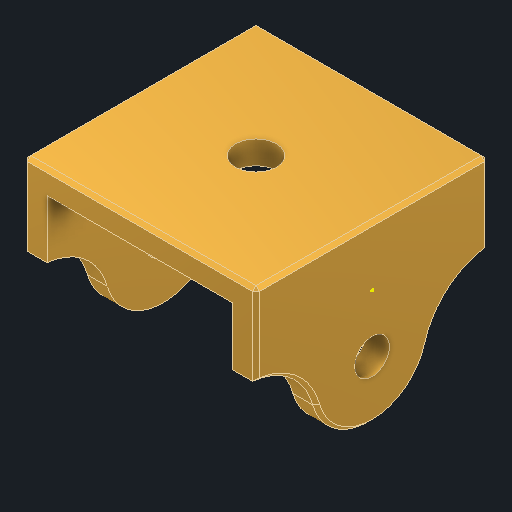
# Autodesk Inventor part: Ball Track Mounting Plate
Saved by Autodesk Inventor 2027.1 (Build 311270010, 270A)
## iProperties
Created: 2025-09-16
Material: Brass, Soft Yellow
Document SubType Name: Modeling
Designer: SD
Density: 8.47 g/cm^3
Appearance: Brass - Satin
Mass: 12.4367 g
Surface Area: 17.3579 cm^2
Volume: 1.46832 cm^3
Project: Automatic Tea Steeping mechanism
Part Number: Ball Track Mounting Plate
d6: 2.000 mm
Length: 20.000 mm
Thickness: 10.000 mm
Width: 20.000 mm
BOM-Mass: 0.01244
BOM-Area: 0.002
Procurement: Fabricate - 2nd round
Build Stage: 3
Preferred Material: C36000 Brass
Author: SD
Title: Ball Track Mounting Plate
Autodesk Inventor part; units mm, degrees
ref_plane "YZ Plane" through (0, 0, 0) normal (1, 0, 0) x (0, 1, 0)
ref_plane "XZ Plane" through (0, 0, 0) normal (0, 1, 0) x (-1, 0, 0)
ref_plane "XY Plane" through (0, 0, 0) normal (0, 0, 1) x (1, 0, 0)
sketch "Sketch1" plane through (0, 0, 0) normal (0, 0, 1) x (1, 0, 0)
  line L0 (-10, 5) -> (10, 5)
  line L1 (10, 5) -> (10, -5)
  line L2 (10, -5) -> (-10, -5)
  line L3 (-10, -5) -> (-10, 5)
  line L4 (-10, 5) -> (10, -5) construction
  line L5 (10, 5) -> (-10, -5) construction
  point P0 (0, 0)
  constraints: 12 end point, 4 parallel, 2 midpoint, 1 horizontal, 1 perpendicular
extrude "Extrusion1" add sketch "Sketch1" along normal mid plane 20
sketch "Sketch3" plane through (10, -5, 10) normal (1, 0, 0) x (0, 0, -1)
  point P0 (10, 5)
sketch "Sketch4" plane through (10, -5, 10) normal (1, 0, 0) x (0, 0, -1)
  line L0 (0, 0) -> (20, 0) projected
  arc A0 (5, 0) -> (15, 0) centre (10, 0) ccw
  point P0 (10, 5)
  dimension "d9" = 10
  constraints: 2 point on circle, 2 point on line, 1 centre point, 1 midpoint
  measures "d9" diameter of A0
extrude "Extrusion3" add sketch "Sketch4" against normal up to surface (20 mm away)
sketch "Sketch2" plane through (0, 0, 10) normal (0, 0, 1) x (1, 0, 0)
  line L0 (-8, -16.4616) -> (8, -16.4616)
  line L1 (8, -16.4616) -> (8, 3)
  line L2 (8, 3) -> (-8, 3)
  line L3 (-8, 3) -> (-8, -16.4616)
  line L4 (-10, 5) -> (-10, -5) projected
  line L5 (10, -5) -> (10, 5) projected
  line L6 (10, 5) -> (-10, 5) projected
  point P0 (0, 0)
  dimension "d4" = 2
  dimension "d5" = 2
  dimension "d6" = 2
  constraints: 8 end point, 2 parallel, 1 horizontal, 1 perpendicular
  measures "d4" distance between parallel lines of L3 L4
  measures "d5" distance between parallel lines of L5 L1
  measures "d6" distance between parallel lines of L2 L6
extrude "Extrusion2" cut sketch "Sketch2" against normal blind 30
sketch "Sketch5" plane through (10, -5, 10) normal (1, 0, 0) x (0, 0, -1)
  line L0 (0, 8) -> (0, 0) projected
  line L1 (5, 0) -> (0, 0) projected
  line L2 (0, 3) -> (5, 3)
  line L3 (5, 3) -> (5, 0)
  line L4 (5, 0) -> (0, 0)
  line L5 (0, 0) -> (0, 3)
  arc A0 (5, 0) -> (15, 0) centre (10, 0) ccw projected
  line L6 (20, 10) -> (20, 0) projected
  line L7 (15, 0) -> (20, 0)
  line L8 (20, 0) -> (20, 3)
  line L9 (20, 3) -> (15, 3)
  line L10 (15, 3) -> (15, 0)
  point P0 (10, 5)
  dimension "d12" = 3
  constraints: 16 end point, 5 parallel, 2 horizontal, 2 perpendicular, 2 point on line
  measures "d12" distance between parallel lines of L1 L2
extrude "Extrusion4" cut sketch "Sketch5" against normal blind 30
fillet "Fillet1" radius 6 4 edges at (9, -2, 5) (9, -2, -5) (-9, -2, 5) (-9, -2, -5)
chamfer "Chamfer1" distance 0.3 angle 45 14 edges at (0, 5, 10) (10, 5, 0) (0, 5, -10) (-10, 5, 0) (-10, 1.5, 10) (10, 1.5, 10) (10, 1.5, -10) (-10, 1.5, -10) (-10, -3.3741, -6.7351) (-10, -10, 0) (-10, -3.3741, 6.7351) (10, -3.3741, -6.7351) (10, -10, 0) (10, -3.3741, 6.7351)
sketch "Sketch6" plane through (-10, -4.2, -14.7) normal (-1, 0, 0) x (0, 0, 1)
  arc A0 (9.8858, -2.1504) -> (19.5142, -2.1504) centre (14.7, -0.8) ccw projected
  circle A1 centre (14.7, -0.8) radius 1.5
  point P0 (14.7, 4.2)
  dimension "d20" = 3
  constraints: 1 centre point, 1 coincident
  measures "d20" diameter of A1
extrude "Extrusion5" cut sketch "Sketch6" against normal blind 30
sketch "Sketch7" plane through (-8, 3, 10) normal (0, -1, 0) x (1, 0, 0)
  point P0 (8, -10)
  point P1 (8, -10)
  constraints: 2 coincident
hole "Hole1" at (0, 3, 0) direction (0, 1, 0) diameter 3.5 depth 11.8 tip angle 118
body "Solid1"
